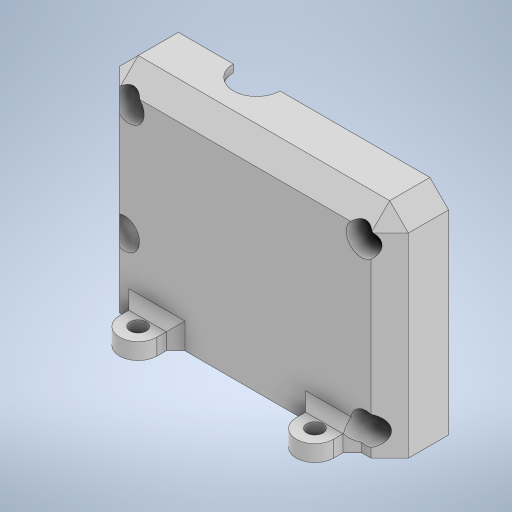
# Autodesk Inventor part: Base_MotorHolder_R
Saved by Autodesk Inventor 2023 (Build 270158000, 158)
## iProperties
Created: 2025-02-06
Part Number: Base_MotorHolder_R
Material: Generic
Document SubType Name: Modeling
Designer: Swoby
Density: 1 g/cm^3
Appearance: Default
Author: Swoby
Autodesk Inventor part; units mm, degrees
ref_plane "YZ Plane" through (0, 0, 0) normal (1, 0, 0) x (0, 1, 0)
ref_plane "XZ Plane" through (0, 0, 0) normal (0, 1, 0) x (-1, 0, 0)
ref_plane "XY Plane" through (0, 0, 0) normal (0, 0, 1) x (1, 0, 0)
sketch "Sketch1" plane through (0, 0, 0) normal (0, 0, 1) x (1, 0, 0)
  line L0 (-20.8, -20.3) -> (20.8, -20.3)
  line L1 (20.8, -20.3) -> (20.8, 20.3)
  line L2 (20.8, 20.3) -> (-20.8, 20.3)
  line L3 (-20.8, 20.3) -> (-20.8, -20.3)
  line L4 (-20.8, -20.3) -> (20.8, 20.3) construction
  line L5 (20.8, -20.3) -> (-20.8, 20.3) construction
  line L6 (-10.15, 10.3885) -> (-10.15, 20.3)
  line L7 (-10.15, 20.3) -> (-17.55, 20.3)
  line L8 (-17.55, 20.3) -> (-17.55, 21.8)
  line L9 (-17.55, 21.8) -> (-10.15, 21.8)
  line L10 (-10.15, 21.8) -> (-10.15, 20.3)
  line L11 (-10.15, 21.8) -> (-15.15, 21.8)
  line L12 (-15.15, 21.8) -> (-15.15, 23.4)
  line L13 (-15.15, 23.4) -> (-10.15, 23.4)
  line L14 (-10.15, 23.4) -> (-10.15, 21.8)
  line L15 (-20.8, 9.1) -> (-27.9, 9.1)
  line L16 (-27.9, 9.1) -> (-27.9, 12.8)
  line L17 (-27.9, 12.8) -> (-20.8, 12.8)
  line L18 (-20.8, 12.8) -> (-20.8, 9.1)
  line L19 (-20.8, -16.4) -> (-30.9, -16.4)
  line L20 (-30.9, -16.4) -> (-30.9, -11)
  line L21 (-30.9, -11) -> (-20.8, -11)
  line L22 (-20.8, -11) -> (-20.8, -16.4)
  line L23 (20.8, 12.8) -> (27.9, 12.8)
  line L24 (27.9, 12.8) -> (27.9, 9.1)
  line L25 (27.9, 9.1) -> (20.8, 9.1)
  line L26 (20.8, 9.1) -> (20.8, 12.8)
  line L27 (-30.9, 23.4) -> (-30.9, -22.3)
  line L28 (-30.9, -22.3) -> (30.9, -22.3)
  line L29 (30.9, -22.3) -> (30.9, 23.4)
  line L30 (-30.9, 23.4) -> (30.9, 23.4)
  point P0 (0, 0)
  point P1 (-15.15, 22.6)
  point P2 (-27.9, 10.95)
  dimension "d0" = 1.5
  dimension "d1" = 1.6
  dimension "d2" = 10.65
  dimension "d4" = 10
  dimension "d5" = 14.8
  dimension "d6" = 7.5
  dimension "d7" = 41.6
  dimension "d8" = 7.1
  dimension "d10" = 7.1
  dimension "d11" = 3.7
  dimension "d12" = 40.6
  dimension "d13" = 3.9
  dimension "d14" = 20.1
  dimension "d15" = 3
  dimension "d16" = 3
  dimension "d17" = 2
  constraints: 62 end point, 12 parallel, 9 perpendicular, 8 point on line, 7 horizontal, 4 midpoint
  measures "d0" distance of L7.end L8.end
  measures "d1" distance of L11.end L12.end
  measures "d2" distance between parallel lines of L3 L10
  measures "d4" diameter of point (-15.15, 22.6) L6
  measures "d5" diameter of L8 L6
  measures "d6" distance between parallel lines of L17 L2
  measures "d7" distance of L1.end L2.end
  measures "d8" distance of L16.end L17.end
  measures "d10" distance of L23.start L23.end
  measures "d11" distance of L15.end L16.end
  measures "d12" distance between parallel lines of L0 L2
  measures "d13" distance between parallel lines of L0 L19
  measures "d14" distance between parallel lines of L21 L15
  measures "d15" distance between parallel lines of L27 L16
  measures "d16" distance between parallel lines of L29 L24
  measures "d17" distance between parallel lines of L28 L0
extrude "Extrusion1" add sketch "Sketch1" against normal blind 10.6 contours L0 L1 L25 L24 L23 L2 L10 L14 L30 L29 L28 L27 L19 L3 | L21 L27 L30 L12 L9 L8 L2 L3 L17 L16 L15 | L2 L8 L9 L10 | L13 L14 L9 L12
revolve "Revolution1" cut sketch "Sketch1" angle 360 about axis through (-10.15, 10.3885, 0) along (0, 1, 0) contours L2 L8 L9 L10 | L13 L14 L9 L12
sketch "Sketch2" plane through (0, 0, -10.6) normal (0, 0, -1) x (-1, 0, 0)
  line L0 (30.9, -11) -> (30.9, 23.4) projected
  line L1 (30.9, 23.4) -> (-30.9, 23.4) projected
  line L2 (-30.9, 23.4) -> (-30.9, -22.3) projected
  line L3 (-30.9, -22.3) -> (30.9, -22.3) projected
  line L4 (30.9, -22.3) -> (30.9, -16.4) projected
  line L5 (30.9, -16.4) -> (20.8, -16.4) projected
  line L6 (20.8, -16.4) -> (20.8, -20.3) projected
  line L7 (20.8, -20.3) -> (-20.8, -20.3) projected
  line L8 (-20.8, -20.3) -> (-20.8, 9.1) projected
  line L9 (-20.8, 9.1) -> (-27.9, 9.1) projected
  line L10 (-27.9, 9.1) -> (-27.9, 12.8) projected
  line L11 (-27.9, 12.8) -> (-20.8, 12.8) projected
  line L12 (-20.8, 12.8) -> (-20.8, 20.3) projected
  line L13 (-20.8, 20.3) -> (20.8, 20.3) projected
  line L14 (20.8, 20.3) -> (20.8, 12.8) projected
  line L15 (20.8, 12.8) -> (27.9, 12.8) projected
  line L16 (27.9, 12.8) -> (27.9, 9.1) projected
  line L17 (27.9, 9.1) -> (20.8, 9.1) projected
  line L18 (20.8, 9.1) -> (20.8, -11) projected
  line L19 (20.8, -11) -> (30.9, -11) projected
  line L20 (30.9, 23.4) -> (-30.9, 23.4)
  line L21 (-30.9, 23.4) -> (-30.9, -22.3)
  line L22 (-30.9, -22.3) -> (30.9, -22.3)
  line L23 (30.9, -22.3) -> (30.9, 23.4)
  point P0 (0, 0)
  constraints: 8 end point, 2 parallel, 1 horizontal, 1 perpendicular
extrude "Extrusion2" add sketch "Sketch2" along normal blind 2
chamfer "Chamfer1" distance 4 angle 45 5 edges at (-30.9, 23.4, -6.3) (-30.9, 0.55, -12.6) (0, 23.4, -12.6) (30.9, 23.4, -6.3) (30.9, 0.55, -12.6)
sketch "Sketch3" plane through (0, 0, 0) normal (0, 0, 1) x (1, 0, 0)
  line L0 (-30.9, 19.4) -> (-26.9, 23.4) projected
  line L1 (-30.9, 19.4) -> (-30.9, -11) projected
  line L2 (-30.9, -11) -> (-20.8, -11) projected
  line L3 (-20.8, -11) -> (-20.8, 9.1) projected
  line L4 (-20.8, 9.1) -> (-27.9, 9.1) projected
  line L5 (-27.9, 9.1) -> (-27.9, 12.8) projected
  line L6 (-27.9, 12.8) -> (-20.8, 12.8) projected
  line L7 (-20.8, 12.8) -> (-20.8, 20.3) projected
  line L8 (-20.8, 20.3) -> (-17.55, 20.3) projected
  line L9 (-17.55, 20.3) -> (-17.55, 21.8) projected
  line L10 (-17.55, 21.8) -> (-15.15, 21.8) projected
  line L11 (-15.15, 21.8) -> (-15.15, 23.4) projected
  line L12 (-15.15, 23.4) -> (-26.9, 23.4) projected
  line L13 (26.9, 23.4) -> (30.9, 19.4) projected
  line L14 (26.9, 23.4) -> (-5.15, 23.4) projected
  line L15 (-5.15, 23.4) -> (-5.15, 21.8) projected
  line L16 (-5.15, 21.8) -> (-2.75, 21.8) projected
  line L17 (-2.75, 21.8) -> (-2.75, 20.3) projected
  line L18 (-2.75, 20.3) -> (20.8, 20.3) projected
  line L19 (20.8, 20.3) -> (20.8, 12.8) projected
  line L20 (20.8, 12.8) -> (27.9, 12.8) projected
  line L21 (27.9, 12.8) -> (27.9, 9.1) projected
  line L22 (27.9, 9.1) -> (20.8, 9.1) projected
  line L23 (20.8, 9.1) -> (20.8, -20.3) projected
  line L24 (20.8, -20.3) -> (-20.8, -20.3) projected
  line L25 (-20.8, -20.3) -> (-20.8, -16.4) projected
  line L26 (-20.8, -16.4) -> (-30.9, -16.4) projected
  line L27 (-30.9, -16.4) -> (-30.9, -22.3) projected
  line L28 (-30.9, -22.3) -> (30.9, -22.3) projected
  line L29 (30.9, -22.3) -> (30.9, 19.4) projected
  line L30 (-20.8, 12.8) -> (-28.9, 21.4) construction
  line L31 (20.8, 12.8) -> (28.9, 21.4) construction
  circle A0 centre (-24.85, 17.1) radius 1.75
  circle A1 centre (24.85, 17.1) radius 1.75
  circle A2 centre (-25.85, -7) radius 1.75
  circle A3 centre (25.85, -17.25) radius 1.75
  point P0 (0, 0)
  dimension "d26" = 3.5
  dimension "d27" = 3.5
  dimension "d28" = 3.5
  dimension "d29" = 3.5
  dimension "d30" = 10.1
  dimension "d31" = 5.05
  dimension "d32" = 5.05
  dimension "d33" = 10.1
  dimension "d34" = 5.05
  dimension "d35" = 4
  constraints: 4 centre point, 4 end point, 4 midpoint
  measures "d26" diameter of A0
  measures "d27" diameter of A1
  measures "d28" diameter of A2
  measures "d29" diameter of A3
  measures "d30" distance between parallel lines of L29 L23
  measures "d31" distance from line of L29 A3.centre
  measures "d32" distance from line of L28 A3.centre
  measures "d33" distance between parallel lines of L1 L3
  measures "d34" distance from line of L3 A2.centre
  measures "d35" distance from line of L2 A2.centre
extrude "Extrusion3" cut sketch "Sketch3" against normal through all contours A0 | A1 | A2 | A3
mirror "Mirror1" about plane through (0, 0.55, 0) normal (0, 0, 1) remove original yes
ref_plane "Work Plane1" through (-15.15, 23.4, 3) normal (0, 0, -1) x (-1, 0, 0)
sketch "Sketch4" plane through (-15.15, 23.4, 3) normal (0, 0, -1) x (-1, 0, 0)
  circle A0 centre (-40, -6.3) radius 1.75 projected
  arc A1 (-42.05, -42.05) -> (-42.05, -39.25) centre (-41, -40.65) ccw projected
  arc A2 (-42.05, -39.25) -> (-42.05, -42.05) centre (-41, -40.65) ccw projected
  circle A3 centre (9.7, -6.3) radius 1.75 projected
  arc A4 (11.75, -29) -> (11.75, -31.8) centre (10.7, -30.4) ccw projected
  arc A5 (11.75, -31.8) -> (11.75, -29) centre (10.7, -30.4) ccw projected
  circle A6 centre (-40, -6.3) radius 3.25
  circle A7 centre (-41, -40.65) radius 3.25
  circle A8 centre (9.7, -6.3) radius 3.25
  circle A9 centre (10.7, -30.4) radius 3.25
  point P0 (-15.15, -23.4)
  dimension "d39" = 6.5
  dimension "d40" = 6.5
  dimension "d41" = 6.5
  dimension "d42" = 6.5
  constraints: 4 centre point, 4 coincident
  measures "d39" diameter of A6
  measures "d40" diameter of A7
  measures "d41" diameter of A8
  measures "d42" diameter of A9
extrude "Extrusion4" cut sketch "Sketch4" against normal through all contours A0 | A2 A1 | A3 | A5 A4 | A6 | A7 | A8 | A9
sketch "Sketch5" plane through (-30.9, -22.3, 0) normal (0, -1, 0) x (1, 0, 0)
  line L0 (61.8, 8.6) -> (57.8, 12.6) projected
  line L1 (57.8, 12.6) -> (4, 12.6) projected
  line L2 (4, 12.6) -> (0, 8.6) projected
  line L3 (0, 0) -> (0, 8.6) projected
  line L4 (0, 0) -> (61.8, 0) projected
  line L5 (61.8, 0) -> (61.8, 8.6) projected
  circle A0 centre (49.8, 16.6) radius 1.75
  arc A1 (53.8, 16.6) -> (45.8, 16.6) centre (49.8, 16.6) ccw
  line L6 (49.8, 16.6) -> (49.8, 12.6) construction
  line L7 (53.8, 16.6) -> (53.8, 12.6)
  line L8 (45.8, 16.6) -> (45.8, 12.6)
  line L9 (30.9, 12.6) -> (30.9, 0) construction
  circle A2 centre (12, 16.6) radius 1.75
  arc A3 (16, 16.6) -> (8, 16.6) centre (12, 16.6) ccw
  line L10 (12, 16.6) -> (12, 12.6) construction
  line L11 (8, 16.6) -> (8, 12.6)
  line L12 (16, 16.6) -> (16, 12.6)
  point P0 (49.8, 14.6)
  point P1 (12, 14.6)
  point P2 (16, 12.6)
  dimension "d45" = 3.5
  dimension "d50" = 4
  dimension "d51" = 12
  dimension "d52" = 4
  constraints: 14 end point, 8 symmetric about line, 4 centre point, 4 point on circle, 3 point on line, 3 vertical, 2 coincident, 2 midpoint, 2 tangent, 1 perpendicular, 2 other
  measures "d45" diameter of A0
  measures "d50" distance of L6.start L6.end
  measures "d51" distance from line of L5 point (49.8, 14.6)
  measures "d52" radius of A1
extrude "Extrusion5" add sketch "Sketch5" against normal blind 3.5 contours L1 L8 A1 L7 | L1 L11 A3 L12
chamfer "Chamfer2" distance 2 angle 45 6 edges at (-22.9, -20.55, 12.6) (-14.9, -20.55, 12.6) (22.9, -20.55, 12.6) (14.9, -20.55, 12.6) (18.9, -18.8, 12.6) (-18.9, -18.8, 12.6)
equation "\"d31\" = 0.5 * d30"
equation "\"d32\" = d31"
equation "\"d34\" = 0.5 * d33"
body "Solid1"
